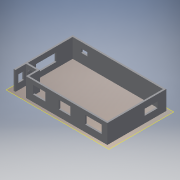
# Autodesk Inventor part: Aussenwand
Saved by Autodesk Inventor 2017 (Build 210142000, 142)
## iProperties
Created: 2017-06-01
Part Number: Aussenwand
Material: Generic
Document SubType Name: Modeling
Designer: Fake
Density: 1 g/cm^3
Appearance: Default
Author: Fake
Autodesk Inventor part; units mm, degrees
ref_plane "YZ Plane" through (0, 0, 0) normal (1, 0, 0) x (0, 1, 0)
ref_plane "XZ Plane" through (0, 0, 0) normal (0, 1, 0) x (-1, 0, 0)
ref_plane "XY Plane" through (0, 0, 0) normal (0, 0, 1) x (1, 0, 0)
ref_plane "Arbeitsebene1" through (0, 0, 1400) normal (0, 0, 1) x (1, 0, 0)
sketch "Skizze1" plane through (0, 0, 1400) normal (0, 0, 1) x (1, 0, 0)
  line L0 (-5480, -3575) -> (-5480, -2375) projected
  line L1 (-5480, -2375) -> (-4200, -2375) projected
  line L2 (-4200, -2375) -> (-4200, -3575) projected
  line L3 (-4200, -3575) -> (5680, -3575) projected
  line L4 (5680, -3575) -> (5680, 3575) projected
  line L5 (5680, 3575) -> (-5680, 3575) projected
  line L6 (-5680, 3575) -> (-5680, -3575) projected
  line L7 (-5680, -3575) -> (-5480, -3575) projected
  line L8 (-5680, 3575) -> (-5680, -3575)
  line L9 (-5480, -3575) -> (-5480, -2275)
  line L10 (-5480, -2275) -> (-4200, -2275)
  line L11 (-4200, -2275) -> (-4200, -3575)
  line L12 (5680, -3575) -> (5680, 3575)
  line L13 (-5680, 3575) -> (5680, 3575)
  line L14 (5680, -3575) -> (-4200, -3575)
  line L15 (-5480, 3375) -> (5480, 3375)
  line L16 (5480, 3375) -> (5480, -3375)
  line L17 (5480, -3375) -> (-4000, -3375)
  line L18 (-4000, -3375) -> (-4000, -2075)
  line L19 (-4000, -2075) -> (-5480, -2075)
  line L20 (-5480, -2075) -> (-5480, 3375)
  line L21 (-5680, -3575) -> (-5480, -3575)
  dimension "d1" = 200
  dimension "d2" = 200
  dimension "d3" = 200
  dimension "d4" = 200
  dimension "d5" = 200
  dimension "d6" = 1300
  dimension "d7" = 200
  constraints: 28 end point, 9 perpendicular, 3 collinear, 2 parallel
  measures "d1" distance between parallel lines of L17 L3
  measures "d2" distance between parallel lines of L18 L2
  measures "d3" distance between parallel lines of L6 L20
  measures "d4" distance between parallel lines of L15 L5
  measures "d5" distance between parallel lines of L4 L16
  measures "d6" distance between parallel lines of L21 L10
  measures "d7" distance between parallel lines of L10 L19
extrude "Extrusion1" add sketch "Skizze1" along normal blind 2300 contours L7 L6 L5 L4 L3 L2 L11 L10 L9 L0
sketch "Skizze2" plane through (-5480, -2275, 1400) normal (0, -1, 0) x (1, 0, 0)
  line L0 (0, 0) -> (1280, 0) projected
  line L1 (1280, 0) -> (1280, 2300) projected
  line L2 (0, 2300) -> (1280, 2300) projected
  line L3 (0, 0) -> (0, 2300) projected
  line L4 (0, 0) -> (1480, 0) projected
  line L5 (156.419, 0) -> (1106.419, 0)
  line L6 (1106.419, 0) -> (1106.419, 1900)
  line L7 (1106.419, 1900) -> (156.419, 1900)
  line L8 (156.419, 1900) -> (156.419, 0)
  dimension "d10" = 950
  dimension "d11" = 1900
  constraints: 8 end point, 2 parallel, 1 horizontal, 1 perpendicular, 1 point on line
  measures "d10" distance of L6.end L7.end
  measures "d11" distance of L7.end L5.start
extrude "Extrusion2" cut sketch "Skizze2" against normal up to surface (200 mm away) contours L8 L7 L6 L0
sketch "Skizze3" plane through (-4200, -3575, 1400) normal (0, -1, 0) x (1, 0, 0)
  line L0 (0, 0) -> (9880, 0) projected
  line L1 (9880, 0) -> (9880, 2300) projected
  line L2 (0, 2300) -> (9880, 2300) projected
  line L3 (0, 0) -> (0, 2300) projected
  line L4 (9175.8648, 1804.3408) -> (7175.8648, 1804.3408)
  line L5 (7175.8648, 1804.3408) -> (7175.8648, 804.3408)
  line L6 (7175.8648, 804.3408) -> (9175.8648, 804.3408)
  line L7 (9175.8648, 804.3408) -> (9175.8648, 1804.3408)
  line L8 (846.0156, 1804.3408) -> (2346.0156, 1804.3408)
  line L9 (2346.0156, 1804.3408) -> (2346.0156, 804.3408)
  line L10 (2346.0156, 804.3408) -> (846.0156, 804.3408)
  line L11 (846.0156, 804.3408) -> (846.0156, 1804.3408)
  line L12 (3985.7595, 1804.3408) -> (5407.0828, 1804.3408)
  line L13 (5407.0828, 1804.3408) -> (5407.0828, 804.3408)
  line L14 (5407.0828, 804.3408) -> (3985.7595, 804.3408)
  line L15 (3985.7595, 804.3408) -> (3985.7595, 1804.3408)
  dimension "d14" = 1000
  dimension "d15" = 2000
  dimension "d22" = 1500
  constraints: 24 end point, 6 parallel, 3 horizontal, 3 perpendicular
  measures "d14" distance of L4.end L5.end
  measures "d15" distance between parallel lines of L7 L5
  measures "d22" distance of L8.start L8.end
extrude "Extrusion3" cut sketch "Skizze3" against normal up to surface (200 mm away) contours L7 L6 L5 L4 | L8 L9 L10 L11 | L12 L13 L14 L15
sketch "Skizze4" plane through (-5680, -3575, 1400) normal (-1, 0, 0) x (0, 0, 1)
  line L0 (0, 7150) -> (0, 0) projected
  line L1 (0, 0) -> (2300, 0) projected
  line L2 (2300, 7150) -> (2300, 0) projected
  line L3 (0, 7150) -> (2300, 7150) projected
  line L4 (1668.3393, 4983.0115) -> (668.3393, 4983.0115)
  line L5 (668.3393, 4983.0115) -> (668.3393, 2483.0115)
  line L6 (668.3393, 2483.0115) -> (1668.3393, 2483.0115)
  line L7 (1668.3393, 2483.0115) -> (1668.3393, 4983.0115)
  line L8 (1668.3393, 338.9652) -> (755.1778, 338.9652)
  line L9 (755.1778, 338.9652) -> (755.1778, 1021.7577)
  line L10 (755.1778, 1021.7577) -> (1668.3393, 1021.7577)
  line L11 (1668.3393, 1021.7577) -> (1668.3393, 338.9652)
  dimension "d18" = 2500
  dimension "d19" = 1000
  constraints: 16 end point, 4 parallel, 2 horizontal, 2 perpendicular
  measures "d18" distance of L6.end L4.start
  measures "d19" distance of L5.end L6.end
extrude "Extrusion4" cut sketch "Skizze4" against normal up to surface (200 mm away) contours L7 L6 L5 L4 | L8 L9 L10 L11
sketch "Skizze5" plane through (5680, -3575, 1400) normal (1, 0, 0) x (0, 0, -1)
  line L0 (-1538.0926, 6113.3523) -> (-798.5727, 6113.3523)
  line L1 (-798.5727, 6113.3523) -> (-798.5727, 4534.3772)
  line L2 (-798.5727, 4534.3772) -> (-1538.0926, 4534.3772)
  line L3 (-1538.0926, 4534.3772) -> (-1538.0926, 6113.3523)
  constraints: 8 end point, 2 parallel, 1 horizontal, 1 perpendicular
extrude "Extrusion5" cut sketch "Skizze5" against normal up to surface (200 mm away)
sketch "Skizze6" plane through (-5680, 3575, 1400) normal (0, 1, 0) x (1, 0, 0)
  line L0 (1998.9049, -1592.9058) -> (1211.657, -1592.9058)
  line L1 (1211.657, -1592.9058) -> (1211.657, -1155.5862)
  line L2 (1211.657, -1155.5862) -> (1998.9049, -1155.5862)
  line L3 (1998.9049, -1155.5862) -> (1998.9049, -1592.9058)
  constraints: 8 end point, 2 parallel, 1 horizontal, 1 perpendicular
extrude "Extrusion6" cut sketch "Skizze6" against normal up to surface (200 mm away)
fillet "Rundung1" radius 470 2 edges at (-5323.581, -2175, 3300) (-4373.581, -2175, 3300)
